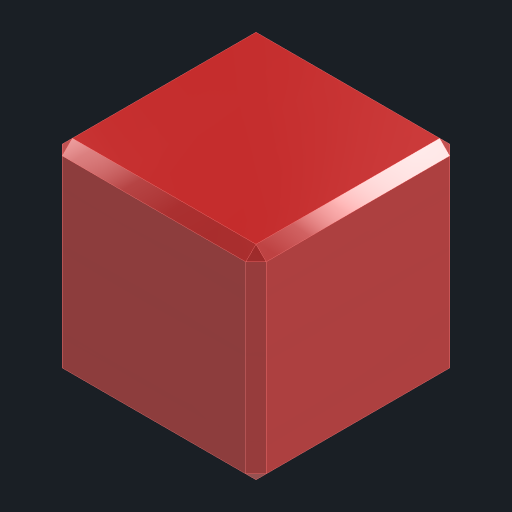
# Autodesk Inventor part: CUBE
Saved by Autodesk Inventor 2023 (Build 270158000, 158)
## iProperties
Created: 2023-03-04
Part Number: CUBE
Material: Generic
Document SubType Name: Modeling
Designer: Phoenix
Density: 1 g/cm^3
Appearance: Red
Author: Phoenix
Autodesk Inventor part; units mm, degrees
ref_plane "YZ Plane" through (0, 0, 0) normal (1, 0, 0) x (0, 1, 0)
ref_plane "XZ Plane" through (0, 0, 0) normal (0, 1, 0) x (-1, 0, 0)
ref_plane "XY Plane" through (0, 0, 0) normal (0, 0, 1) x (1, 0, 0)
sketch "Sketch1" plane through (0, 0, 0) normal (0, 1, 0) x (-1, 0, 0)
  line L0 (0, 0) -> (-40, 0)
  line L1 (-40, 0) -> (-40, 40)
  line L2 (-40, 40) -> (0, 40)
  line L3 (0, 40) -> (0, 0)
  dimension "d0" = 40
  dimension "d1" = 40
  constraints: 8 end point, 2 parallel, 1 horizontal, 1 perpendicular
  measures "d0" distance of L1.end L2.end
  measures "d1" distance of L0.end L1.end
extrude "Extrusion1" add sketch "Sketch1" along normal blind 40
chamfer "Chamfer1" distance 2 angle 45 12 edges at (20, 0, 40) (40, 0, 20) (20, 40, 0) (20, 0, 0) (0, 20, 0) (0, 40, 20) (0, 20, 40) (0, 0, 20) (20, 40, 40) (40, 20, 40) (40, 40, 20) (40, 20, 0)
equation "\"d0\" = CUBE_D"
equation "\"d1\" = CUBE_D"
equation "\"d2\" = CUBE_D"
equation "\"CUBE_D\" = 40"
body "Solid1"
